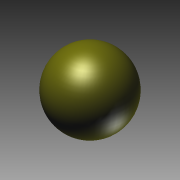
# Autodesk Inventor part: W 638/4 XR-2Z_PART3
Saved by Autodesk Inventor 2011 SP1 (Build 150282100, 282)
## iProperties
Created: 2017-05-31
Part Number: W 638/4 XR-2Z_PART3
Catalog Web Link: www.cadenas.de
Description: -Deep groove ball bearings, stainless steel, single row, with flanged outer ring
Vendor: SKF
Document SubType Name: Modeling
Designer: psAdmin
Manufacturer: SKF
Mass: 0.00209677 g
Surface Area: 0.0792229 cm^2
Volume: 0.00209677 cm^3
Density: 1 g/cm^3
Category: PARTsolutions
Company: SKF
Title: W 638/4 XR-2Z_PART3
Author: Cadenas PARTsolutions
Comments: Deep groove ball bearings, stainless steel, single row, with flanged outer ring
PSOL_IDENT_0: {$CADENAS_DATA\23d-libs\skf\bearings_units_and_housings\ball_bearings\deep_groove_ball_bearings\deep
PSOL_IDENT_1: _groove_ball_bearings_stainless_steel\bb1_005_105.prj},207 {VTYP=3D},{NB=W 638/4 XR-2Z_PART3},{LINA=
PSOL_IDENT_2: W 638/4 XR-2Z_PART3},{NN=BB1_005_105_PART3},{NOPRJ=TRUE},{DATE=12.09.2016 08:57:11},{GEOMDATE=26.04.
PSOL_IDENT_3: 2016 08:41:00},{VERSION=},{LINEID=51210},{LINESUBID=-1},{WBVAR=}  {NB=W 638/4 XR-2Z_PART3},{LINA=W 6
PSOL_IDENT_4: 38/4 XR-2Z_PART3},{KT=DUMMY},{PRODUCTID=},{DESIGNATION=W 638/4 XR-2Z},{DD=4.000},{D=10.000},{B=4.000
PSOL_IDENT_5: },{C=0.800},{DD1=5.900},{DD2=-1000000015047466219876688855040.000},{D1=8.200},{D2=8.800},{D3=11.600}
PSOL_IDENT_6: ,{R12=0.150},{LOAD1=0.553},{LOAD2=0.245},{LOAD3=0.011},{SPEED1=130000},{SPEED2=63000},{MASS=0.0015},
PSOL_IDENT_7: {PITCH=7.100},{DW=1.588},{Z=8.000},{II=1.000},{TYPEID=-1000000015047466219876688855040},{DESIGN=dgbb
PSOL_IDENT_8: wr2z},{MAPPING=BCZ50,DESIGNATION|IRD01,DD|ORD10,D|BCW30,B|ORL02,C|IRD30,DD1|ORD30,D1|IRD43,DD2|ORD43
PSOL_IDENT_9: ,D2|ORD15,D3|ORR20,R12|BCC02,LOAD1|BCC16,LOAD2|BCC12,LOAD3|BCC43,SPEED1|BCC45,SPEED2|BCM01,MASS|BCD5
PSOL_IDENT_10: 0,PITCH|RBD10,DW|BCN81,Z|BCN80,II},{DESIGNLIST=dgbbwr2rs,dgbbwr,dgbbwr2z,dgbbwr2rz,dgbbwr2zs},{SORT=
PSOL_IDENT_11: DD},{SH=5.9},{PIM=W 638/4 XR-2Z}
NT: Deep groove ball bearings, stainless steel, single row, with flanged outer ring
NB: W 638/4 XR-2Z_PART3
NBSYN: $DESIGNATION._PART3
LINA: W 638/4 XR-2Z_PART3
DESIGNATION: W 638/4 XR-2Z
DD: 4.000
D: 10.000
B: 4.000
LOAD1: 0.553
LOAD2: 0.245
LOAD3: 0.011
SPEED1: 130000
SPEED2: 63000
SUPPLIER: SKF
ARTICLENO: W 638/4 XR-2Z_PART3
BOMINFO: W 638/4 XR-2Z_PART3
CREATOR: CADENAS GmbH
Autodesk Inventor part; units mm, degrees
ref_plane "YZ Plane" through (0, 0, 0) normal (1, 0, 0) x (0, 1, 0)
ref_plane "XZ Plane" through (0, 0, 0) normal (0, 1, 0) x (-1, 0, 0)
ref_plane "XY Plane" through (0, 0, 0) normal (0, 0, 1) x (1, 0, 0)
sketch "Sketch_4" plane through (0, 0, 0) normal (0, 0, 1) x (1, 0, 0)
  line L0 (2.794, 3.55) -> (1.206, 3.55)
  arc A0 (2.794, 3.55) -> (1.206, 3.55) centre (2, 3.55) ccw
  line L1 (2.794, 3.55) -> (1.206, 3.55)
  dimension "d0" = 360
  constraints: 4 end point, 2 point on circle, 1 centre point
revolve "Revolution1" add sketch "Sketch_4" angle 360 about axis through (2.794, 3.55, 0) along (1, 0, 0)
body "Solid1"
